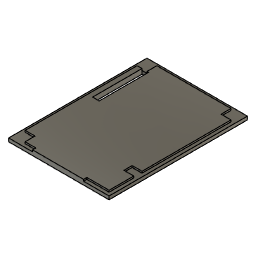
RB_STM32_DVM_4_Lid v1 (Autodesk Fusion 360 design; units mm, degrees)
Autodesk Fusion 360 part; units mm, degrees
sketch "Sketch1" plane through (0, 0, 0) normal (0, 0, 1) x (1, 0, 0)
  line L0 (0, 0) -> (61, 0)
  line L1 (61, 0) -> (61, 84)
  line L2 (61, 84) -> (0, 84)
  line L3 (0, 84) -> (0, 0)
  dimension "d1" = 61
  dimension "d2" = 84
  constraint horizontal L0
  constraint vertical L1
  constraint horizontal L2
  constraint vertical L3
  constraint coincident L0.start L3.end
  measures "d1" distance of L0.start L0.end
  measures "d2" distance of L0.start L2.end
extrude "Extrude1" add sketch "Sketch1" along normal blind 2
sketch "Sketch2" plane through (0, 0, 2) normal (0, 0, 1) x (-1, 0, 0)
  line L0 (0, -84) -> (0, 0)
  line L1 (0, 0) -> (-61, 0)
  line L2 (-61, 0) -> (-61, -84)
  line L3 (-61, -84) -> (0, -84)
  line L4 (-2, -2) -> (-59, -2)
  line L5 (-59, -2) -> (-59, -82)
  line L6 (-59, -82) -> (-2, -82)
  line L7 (-2, -82) -> (-2, -2)
  dimension "d5" = 57
  dimension "d6" = 80
  constraint horizontal L4
  constraint vertical L5
  constraint horizontal L6
  constraint vertical L7
  measures "d5" distance of L4.start L4.end
  measures "d6" distance of L4.start L6.end
extrude "Extrude2" add sketch "Sketch2" along normal blind 1 contours L4 L5 L6 L7
sketch "Sketch3" plane through (0, 0, 3) normal (0, 0, 1) x (-1, 0, 0)
  line L0 (-2, -82) -> (-2, -2)
  line L1 (-2, -2) -> (-59, -2)
  line L2 (-59, -2) -> (-59, -82)
  line L3 (-59, -82) -> (-2, -82)
  line L4 (-59, -82) -> (-53, -82)
  line L5 (-53, -82) -> (-53, -76)
  line L6 (-53, -76) -> (-59, -76)
  line L7 (-59, -76) -> (-59, -82)
  constraint horizontal L4
  constraint vertical L5
  constraint horizontal L6
  constraint vertical L7
  constraint coincident L2.end L3.start
extrude "Extrude3" cut sketch "Sketch3" against normal blind 1 contours L2 L3 L4 L5 L6 L7
sketch "Sketch4" plane through (0, 0, 3) normal (0, 0, 1) x (-1, 0, 0)
  line L0 (-53, -76) -> (-53, -82)
  line L1 (-53, -82) -> (-2, -82)
  line L2 (-2, -82) -> (-2, -2)
  line L3 (-2, -2) -> (-59, -2)
  line L4 (-59, -2) -> (-59, -76)
  line L5 (-59, -76) -> (-53, -76)
  line L6 (-2, -82) -> (-8, -82)
  line L7 (-8, -82) -> (-8, -76)
  line L8 (-8, -76) -> (-2, -76)
  line L9 (-2, -76) -> (-2, -82)
  constraint horizontal L6
  constraint vertical L7
  constraint horizontal L8
  constraint vertical L9
  constraint coincident L1.end L2.start
extrude "Extrude4" cut sketch "Sketch4" against normal blind 1 contours L1 L2 L6 L7 L8 L9
sketch "Sketch5" plane through (0, 0, 3) normal (0, 0, 1) x (-1, 0, 0)
  line L0 (-8, -76) -> (-2, -76)
  line L1 (-2, -76) -> (-2, -2)
  line L2 (-2, -2) -> (-59, -2)
  line L3 (-59, -2) -> (-59, -76)
  line L4 (-59, -76) -> (-53, -76)
  line L5 (-53, -76) -> (-53, -82)
  line L6 (-53, -82) -> (-8, -82)
  line L7 (-8, -82) -> (-8, -76)
  line L8 (-2, -2) -> (-8, -2)
  line L9 (-8, -2) -> (-8, -8)
  line L10 (-8, -8) -> (-2, -8)
  line L11 (-2, -8) -> (-2, -2)
  constraint horizontal L8
  constraint vertical L9
  constraint horizontal L10
  constraint vertical L11
  constraint coincident L1.end L2.start
extrude "Extrude5" cut sketch "Sketch5" against normal blind 1 contours L1 L2 L8 L9 L10 L11
sketch "Sketch6" plane through (0, 0, 2) normal (0, 0, 1) x (-1, 0, 0)
  line L0 (-8, -82) -> (-53, -82)
  line L1 (-53, -82) -> (-53, -76)
  line L2 (-53, -76) -> (-59, -76)
  line L3 (-59, -76) -> (-59, -2)
  line L4 (-59, -2) -> (-8, -2)
  line L5 (-8, -2) -> (-8, -8)
  line L6 (-8, -8) -> (-2, -8)
  line L7 (-2, -8) -> (-2, -76)
  line L8 (-2, -76) -> (-8, -76)
  line L9 (-8, -76) -> (-8, -82)
  line L10 (0, -84) -> (0, 0)
  line L11 (0, 0) -> (-61, 0)
  line L12 (-61, 0) -> (-61, -84)
  line L13 (-61, -84) -> (0, -84)
  line L14 (-14.5, 0) -> (-45.5, 0)
  line L15 (-45.5, 0) -> (-45.5, -2)
  line L16 (-45.5, -2) -> (-14.5, -2)
  line L17 (-14.5, -2) -> (-14.5, 0)
  dimension "d15" = 31
  dimension "d16" = 2
  constraint horizontal L14
  constraint vertical L15
  constraint horizontal L16
  constraint vertical L17
  constraint coincident L11 L14.start
  measures "d15" distance of L14.start L14.end
  measures "d16" distance of L14.start L16.end
extrude "Extrude6" add sketch "Sketch6" along normal blind 1 contours L4 L11 L14 L15 L16 L17
sketch "Sketch7" plane through (0, 0, 3) normal (0, 0, 1) x (-1, 0, 0)
  line L0 (-8, -8) -> (-8, -2)
  line L1 (-8, -2) -> (-14.5, -2)
  line L2 (-14.5, -2) -> (-14.5, 0)
  line L3 (-14.5, 0) -> (-45.5, 0)
  line L4 (-45.5, 0) -> (-45.5, -2)
  line L5 (-45.5, -2) -> (-59, -2)
  line L6 (-59, -2) -> (-59, -76)
  line L7 (-59, -76) -> (-53, -76)
  line L8 (-53, -76) -> (-53, -82)
  line L9 (-53, -82) -> (-8, -82)
  line L10 (-8, -82) -> (-8, -76)
  line L11 (-8, -76) -> (-2, -76)
  line L12 (-2, -76) -> (-2, -8)
  line L13 (-2, -8) -> (-8, -8)
  line L14 (-53, -17) -> (-59, -17)
  line L15 (-59, -17) -> (-59, -22)
  line L16 (-59, -22) -> (-53, -22)
  line L17 (-53, -22) -> (-53, -17)
  dimension "d19" = 5
  constraint horizontal L14
  constraint vertical L15
  constraint horizontal L16
  constraint vertical L17
  measures "d19" distance of L14.start L16.end
extrude "Extrude7" cut sketch "Sketch7" against normal blind 1 contours L6 L14 L15 L16 L17
sketch "Sketch8" plane through (0, 0, 3) normal (0, 0, 1) x (-1, 0, 0)
  line L0 (-53, -22) -> (-59, -22)
  line L1 (-59, -22) -> (-59, -76)
  line L2 (-59, -76) -> (-53, -76)
  line L3 (-53, -76) -> (-53, -82)
  line L4 (-53, -82) -> (-8, -82)
  line L5 (-8, -82) -> (-8, -76)
  line L6 (-8, -76) -> (-2, -76)
  line L7 (-2, -76) -> (-2, -8)
  line L8 (-2, -8) -> (-8, -8)
  line L9 (-8, -8) -> (-8, -2)
  line L10 (-8, -2) -> (-14.5, -2)
  line L11 (-14.5, -2) -> (-14.5, 0)
  line L12 (-14.5, 0) -> (-45.5, 0)
  line L13 (-45.5, 0) -> (-45.5, -2)
  line L14 (-45.5, -2) -> (-59, -2)
  line L15 (-59, -2) -> (-59, -17)
  line L16 (-59, -17) -> (-53, -17)
  line L17 (-53, -17) -> (-53, -22)
  line L18 (-5, -76) -> (-9, -76)
  line L19 (-9, -76) -> (-9, -46)
  line L20 (-9, -46) -> (-5, -46)
  line L21 (-5, -46) -> (-5, -76)
  dimension "d22" = 4
  dimension "d23" = 30
  constraint horizontal L18
  constraint vertical L19
  constraint horizontal L20
  constraint vertical L21
  constraint midpoint L6 L18.start
  measures "d22" distance of L18.start L18.end
  measures "d23" distance of L18.start L20.end
extrude "Extrude8" cut sketch "Sketch8" against normal blind 4 contours L6 L18 L19 L20 L21
